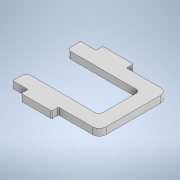
# Autodesk Inventor part: Laser-Slot-Endstop
Saved by Autodesk Inventor 2021 (Build 250183000, 183)
## iProperties
Created: 2020-08-04
Part Number: Laser-Slot-Endstop
Material: Generic
Document SubType Name: Modeling
Designer: lucas
Density: 1 g/cm^3
Appearance: Default
Project: 4Wire-Laser
Author: lucas
Revision Number: RLS_001
Autodesk Inventor part; units mm, degrees
ref_plane "YZ Plane" through (0, 0, 0) normal (1, 0, 0) x (0, 1, 0)
ref_plane "XZ Plane" through (0, 0, 0) normal (0, 1, 0) x (-1, 0, 0)
ref_plane "XY Plane" through (0, 0, 0) normal (0, 0, 1) x (1, 0, 0)
sketch "Sketch1" plane through (0, 0, 0) normal (0, 1, 0) x (-1, 0, 0)
  line L0 (-9, 0) -> (-19, 0)
  line L1 (-21, -2) -> (-21, -18)
  line L2 (-19, -20) -> (-9, -20)
  line L3 (0, -20) -> (2, -20)
  line L4 (0, 0) -> (2, 0)
  line L5 (-9, 0) -> (-9, 2)
  line L6 (-9, 2) -> (0, 2)
  line L7 (0, 2) -> (0, 0)
  line L8 (-9, -20) -> (-9, -22)
  line L9 (-9, -22) -> (0, -22)
  line L10 (0, -22) -> (0, -20)
  line L11 (2, 0) -> (2, -3)
  line L12 (1, -4) -> (-15.9, -4)
  line L13 (-16.9, -5) -> (-16.9, -15)
  line L14 (-15.9, -16) -> (1, -16)
  line L15 (2, -17) -> (2, -20)
  arc A0 (1, -4) -> (2, -3) centre (1, -3) ccw
  arc A1 (2, -17) -> (1, -16) centre (1, -17) ccw
  arc A2 (-15.9, -4) -> (-16.9, -5) centre (-15.9, -5) ccw
  arc A3 (-16.9, -15) -> (-15.9, -16) centre (-15.9, -15) ccw
  arc A4 (-21, -18) -> (-19, -20) centre (-19, -18) ccw
  arc A5 (-19, 0) -> (-21, -2) centre (-19, -2) ccw
  line L16 (2, 0) -> (4.5, 0)
  line L17 (4.5, 0) -> (4.5, -3)
  line L18 (3.5, -4) -> (1, -4)
  line L19 (2, -20) -> (4.5, -20)
  line L20 (4.5, -20) -> (4.5, -17)
  line L21 (3.5, -16) -> (1, -16)
  arc A6 (3.5, -4) -> (4.5, -3) centre (3.5, -3) ccw
  arc A7 (4.5, -17) -> (3.5, -16) centre (3.5, -17) ccw
  point P0 (-21, 0)
  point P1 (-21, -20)
  point P2 (2, -4)
  point P3 (-16.9, -4)
  point P4 (-16.9, -16)
  point P5 (2, -16)
  point P6 (4.5, -16)
  dimension "d1" = 12
  dimension "d5" = 2
  dimension "d6" = 2
  dimension "d7" = 2
  dimension "d8" = 2
  dimension "d9" = 4
  dimension "d11" = 12
  dimension "d12" = 9
  dimension "d13" = 9
  dimension "d14" = 1
  dimension "d17" = 18.9
  dimension "d18" = 20
  dimension "d19" = 2
  dimension "d20" = 2.5
  dimension "d21" = 1
  constraints: 44 end point, 21 point on line, 17 tangent, 16 point on circle, 8 centre point, 8 perpendicular, 5 equal radius, 3 equal length, 3 horizontal, 2 parallel, 1 vertical
  measures "d1" distance of L0.start point (-21, 0)
  measures "d5" distance of L3.start L3.end
  measures "d6" distance of L4.start L4.end
  measures "d7" distance of L0.start L5.end
  measures "d8" distance of L2.end L8.end
  measures "d9" distance of L4.end point (2, -4)
  measures "d11" distance of point (-16.9, -4) point (-16.9, -16)
  measures "d12" distance of L5.end L6.end
  measures "d13" distance of L8.end L9.end
  measures "d14" radius of A0
  measures "d17" distance between parallel lines of L13 L11
  measures "d18" distance between parallel lines of L2 L0
  measures "d19" radius of A4
  measures "d20" distance of L4.end L16.end
  measures "d21" radius of A6
extrude "Extrusion1" add sketch "Sketch1" along normal blind 2
fillet "Fillet1" radius 0.25 10 edges at (9, 1, 0) (9, 1, 2) (0, 1, 2) (0, 1, 0) (9, 1, -20) (9, 1, -22) (0, 1, -22) (0, 1, -20) (-4.5, 1, 0) (-4.5, 1, -20)
body "Solid1"
